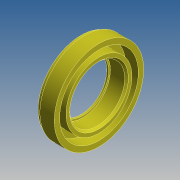
# Autodesk Inventor part: P114PorteLentille20mm
Saved by Autodesk Inventor 2015 SP1 (Build 190203100, 203)
## iProperties
Created: 2016-11-02
Part Number: P114PorteLentille20mm
Material: ABS Plastic
Document SubType Name: Modeling
Designer: serge.amoos
Density: 1.06 g/cm^3
Appearance: Canary
Author: serge.amoos
Autodesk Inventor part; units mm, degrees
ref_plane "YZ Plane" through (0, 0, 0) normal (1, 0, 0) x (0, 1, 0)
ref_plane "XZ Plane" through (0, 0, 0) normal (0, 1, 0) x (-1, 0, 0)
ref_plane "XY Plane" through (0, 0, 0) normal (0, 0, 1) x (1, 0, 0)
sketch "Sketch1" plane through (0, 0, 0) normal (0, 0, 1) x (1, 0, 0)
  line L0 (-12, 0) -> (2, 0) construction
  line L1 (0, -4.98) -> (0, 29.88) construction
  line L2 (0, 15.35) -> (-9, 15.35)
  line L3 (-9, 15.35) -> (-9, 14.35)
  line L4 (-9, 14.35) -> (-10, 14.35)
  line L5 (-10, 14.35) -> (-10, 23.9)
  line L6 (-10, 23.9) -> (-8, 23.9)
  line L7 (-8, 23.9) -> (-8, 24.9)
  line L8 (-8, 24.9) -> (0, 24.9)
  line L9 (0, 21.9) -> (-7, 21.9)
  line L10 (-7, 21.9) -> (-7, 18.35)
  line L11 (-7, 18.35) -> (0, 18.35)
  line L12 (0, 24.9) -> (0, 21.9)
  line L13 (0, 18.35) -> (0, 15.35)
  point P0 (0, 0)
  dimension "d0" = 49.8
  dimension "d1" = 47.8
  dimension "d3" = 1
  dimension "d4" = 2
  dimension "d5" = 30.7
  dimension "d6" = 1
  dimension "d7" = 3
  dimension "d8" = 3
  dimension "d9" = 3
  dimension "d10" = 10
  constraints: 24 end point, 9 perpendicular, 2 collinear, 2 point on line, 1 horizontal
  measures "d0" diameter of L8 L0
  measures "d1" diameter of L6 L0
  measures "d3" distance between parallel lines of L3 L5
  measures "d4" distance between parallel lines of L5 L7
  measures "d5" diameter of L2 L0
  measures "d6" distance of L2.end L3.end
  measures "d7" distance between parallel lines of L9 L8
  measures "d8" distance between parallel lines of L10 L5
  measures "d9" distance between parallel lines of L2 L11
  measures "d10" distance between parallel lines of L1 L5
revolve "Revolution1" add sketch "Sketch1" angle 360 about axis through (-10, 0, 0) along (1, 0, 0)
chamfer "Chamfer1" distance 1 angle 45 1 edges at (0, -15.35, 0)
body "Solid1"
